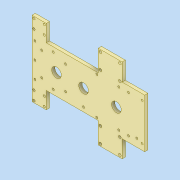
# Autodesk Inventor part: 底盘4.0
Saved by Autodesk Inventor 2019 (Build 230136000, 136)
## iProperties
Created: 2020-11-02
Part Number: 底盘4.0
Material: 尼龙 6/6
Document SubType Name: Modeling
Designer: Wang Hua
Density: 1.13 g/cm^3
Appearance: 尼龙 6
Mass: 59.1636 g
Surface Area: 303.115 cm^2
Volume: 52.3571 cm^3
Author: Wang Hua
Autodesk Inventor part; units mm, degrees
ref_plane "YZ Plane" through (0, 0, 0) normal (1, 0, 0) x (0, 1, 0)
ref_plane "XZ Plane" through (0, 0, 0) normal (0, 1, 0) x (-1, 0, 0)
ref_plane "XY Plane" through (0, 0, 0) normal (0, 0, 1) x (1, 0, 0)
sketch "草图1" plane through (0, 0, 0) normal (0, 0, 1) x (1, 0, 0)
  line L0 (-144.4444, 0) -> (-144.4444, 58)
  line L1 (-144.4444, 58) -> (-122.4444, 58)
  line L2 (-122.4444, 58) -> (-122.4444, 32)
  line L3 (-122.4444, 32) -> (-41.9444, 32)
  line L4 (-41.9444, 32) -> (-41.9444, 65)
  line L5 (-41.9444, 65) -> (-4.9444, 65)
  line L6 (-4.9444, 65) -> (-4.9444, 38)
  line L7 (-4.9444, 38) -> (30.0556, 38)
  line L8 (30.0556, 38) -> (30.0556, 0)
  line L9 (0, 0) -> (-166.6667, 0) construction
  line L10 (-144.4444, 0) -> (-144.4444, -58)
  line L11 (-144.4444, -58) -> (-122.4444, -58)
  line L12 (-122.4444, -58) -> (-122.4444, -32)
  line L13 (-122.4444, -32) -> (-41.9444, -32)
  line L14 (-41.9444, -32) -> (-41.9444, -65)
  line L15 (-41.9444, -65) -> (-4.9444, -65)
  line L16 (-4.9444, -65) -> (-4.9444, -38)
  line L17 (-4.9444, -38) -> (30.0556, -38)
  line L18 (30.0556, -38) -> (30.0556, 0)
  circle A0 centre (-106.5528, 0) radius 7.5
  circle A1 centre (-64.5976, 0) radius 7.5
  point P0 (-141.4444, -54)
  point P1 (-127.4444, -54)
  point P2 (-27.9137, -54)
  point P3 (-14.1378, -54)
  point P4 (-112.1204, -28)
  point P5 (-64.5976, -28)
  point P6 (-89.6514, -28)
  point P7 (-127.4444, -38)
  point P8 (-141.4444, -38)
  point P9 (-27.9137, -38)
  point P10 (-14.3619, -38)
  point P11 (-141.4444, 54)
  point P12 (-127.4444, 54)
  point P13 (-127.4444, 38)
  point P14 (-141.4444, 38)
  point P15 (-27.9137, 54)
  point P16 (-27.9137, 38)
  point P17 (-14.1378, 54)
  point P18 (-14.3619, 38)
  point P19 (-64.5976, 28)
  point P20 (-89.6514, 28)
  point P21 (-112.1204, 28)
  point P22 (-133.4444, 58)
  point P23 (-23.4444, 65)
  dimension "d0" = 22
  dimension "d1" = 37
  dimension "d3" = 32
  dimension "d4" = 38
  dimension "d5" = 35
  dimension "d6" = 58
  dimension "d7" = 15
  dimension "d8" = 15
  dimension "d29" = 28
  dimension "d30" = 28
  dimension "d31" = 28
  dimension "d36" = 110
  dimension "d96" = 33
  constraints: 38 end point, 19 symmetric about line, 5 perpendicular, 4 point on line, 2 centre point, 2 midpoint, 2 vertical, 1 horizontal
  measures "d0" distance of L0.end L1.end
  measures "d1" distance of L4.end L5.end
  measures "d3" distance between parallel lines of L9 L3
  measures "d4" distance between parallel lines of L9 L7
  measures "d5" distance of L6.end L7.end
  measures "d6" distance of L0.start L0.end
  measures "d7" diameter of A0
  measures "d8" diameter of A1
  measures "d29" distance from line of L9 point (-112.12, 28)
  measures "d30" distance from line of L9 point (-89.651, 28)
  measures "d31" distance from line of L9 point (-64.598, 28)
  measures "d36" horizontal distance of point (-23.444, 65) point (-133.444, 58)
  measures "d96" distance between parallel lines of L5 L3
extrude "拉伸1" add sketch "草图1" along normal blind 5
sketch "草图2" plane through (0, 0, 5) normal (0, 0, 1) x (1, 0, 0)
  circle A0 centre (-64.5976, 0) radius 7.5 construction
  circle A1 centre (-106.5528, 0) radius 7.5 construction
  line L0 (-144.4444, -58) -> (-144.4444, 58) construction
  line L1 (-144.4444, 58) -> (-122.4444, 58) construction
  line L2 (-122.4444, 58) -> (-122.4444, 32) construction
  line L3 (-122.4444, 32) -> (-41.9444, 32) construction
  line L4 (-41.9444, 32) -> (-41.9444, 65) construction
  line L5 (-41.9444, 65) -> (-4.9444, 65) construction
  line L6 (-4.9444, 65) -> (-4.9444, 38) construction
  line L7 (-4.9444, 38) -> (30.0556, 38) construction
  line L8 (30.0556, 38) -> (30.0556, -38) construction
  line L9 (30.0556, -38) -> (-4.9444, -38) construction
  line L10 (-4.9444, -38) -> (-4.9444, -65) construction
  line L11 (-4.9444, -65) -> (-41.9444, -65) construction
  line L12 (-41.9444, -65) -> (-41.9444, -32) construction
  line L13 (-41.9444, -32) -> (-122.4444, -32) construction
  line L14 (-122.4444, -32) -> (-122.4444, -58) construction
  line L15 (-122.4444, -58) -> (-144.4444, -58) construction
  line L16 (-164.7255, 0) -> (-80.9793, 0) construction
  point P0 (0, 0)
  point P1 (-141.4444, 55)
  point P2 (-125.4444, 55)
  point P3 (-38.4444, 61.5)
  point P4 (-8.4444, 61.5)
  point P5 (-38.4444, 37.5)
  point P6 (-8.4444, 37.5)
  point P7 (-125.4444, 41)
  point P8 (-141.4444, 41)
  point P9 (-141.4444, -55)
  point P10 (-125.4444, -55)
  point P11 (-38.4444, -61.5)
  point P12 (-8.4444, -61.5)
  point P13 (-38.4444, -37.5)
  point P14 (-8.4444, -37.5)
  point P15 (-125.4444, -41)
  point P16 (-141.4444, -41)
  dimension "d32" = 3
  dimension "d33" = 3
  dimension "d34" = 16
  dimension "d37" = 3
  dimension "d38" = 14
  dimension "d39" = 3
  dimension "d40" = 14
  dimension "d42" = 30
  dimension "d43" = 30
  dimension "d44" = 24
  dimension "d45" = 3.5
  dimension "d46" = 3.5
  dimension "d47" = 3.5
  dimension "d95" = 16
  constraints: 8 symmetric about line, 2 end point, 1 horizontal
  measures "d32" distance from line of L1 point (-125.444, 55)
  measures "d33" distance from line of L1 point (-141.444, 55)
  measures "d34" distance of point (-125.444, 55) point (-141.444, 55)
  measures "d37" distance from line of L0 point (-141.444, 55)
  measures "d38" distance of point (-141.444, 55) point (-141.444, 41)
  measures "d39" distance from line of L0 point (-141.444, 41)
  measures "d40" distance of point (-125.444, 55) point (-125.444, 41)
  measures "d42" distance of point (-8.444, 61.5) point (-38.444, 61.5)
  measures "d43" distance of point (-8.444, 37.5) point (-38.444, 37.5)
  measures "d44" distance of point (-38.444, 61.5) point (-38.444, 37.5)
  measures "d45" distance from line of L5 point (-38.444, 61.5)
  measures "d46" distance from line of L4 point (-38.444, 37.5)
  measures "d47" distance from line of L4 point (-38.444, 61.5)
  measures "d95" distance of point (-141.444, 41) point (-125.444, 41)
hole "孔2" at (-141.4444, 55, 5) at (-125.4444, 55, 5) at (-125.4444, 41, 5) at (-141.4444, 41, 5) at (-141.4444, -41, 5) at (-125.4444, -41, 5) at (-125.4444, -55, 5) at (-141.4444, -55, 5) direction (0, 0, -1) diameter 3.6 end through all
sketch "草图3" plane through (0, 0, 5) normal (0, 0, 1) x (1, 0, 0)
  circle A0 centre (-125.4444, -55) radius 1.8 construction
  circle A1 centre (-141.4444, -55) radius 1.8 construction
  circle A2 centre (-125.4444, 41) radius 1.8 construction
  circle A3 centre (-141.4444, 55) radius 1.8 construction
  circle A4 centre (-125.4444, 55) radius 1.8 construction
  circle A5 centre (-141.4444, 41) radius 1.8 construction
  circle A6 centre (-141.4444, -41) radius 1.8 construction
  circle A7 centre (-125.4444, -41) radius 1.8 construction
  circle A8 centre (-64.5976, 0) radius 7.5 construction
  circle A9 centre (-106.5528, 0) radius 7.5 construction
  line L0 (-144.4444, 58) -> (-144.4444, -58) construction
  line L1 (-144.4444, -58) -> (-122.4444, -58) construction
  line L2 (-122.4444, -58) -> (-122.4444, -32) construction
  line L3 (-122.4444, -32) -> (-41.9444, -32) construction
  line L4 (-41.9444, -32) -> (-41.9444, -65) construction
  line L5 (-41.9444, -65) -> (-4.9444, -65) construction
  line L6 (-4.9444, -65) -> (-4.9444, -38) construction
  line L7 (-4.9444, -38) -> (30.0556, -38) construction
  line L8 (30.0556, -38) -> (30.0556, 38) construction
  line L9 (30.0556, 38) -> (-4.9444, 38) construction
  line L10 (-4.9444, 38) -> (-4.9444, 65) construction
  line L11 (-4.9444, 65) -> (-41.9444, 65) construction
  line L12 (-41.9444, 65) -> (-41.9444, 32) construction
  line L13 (-41.9444, 32) -> (-122.4444, 32) construction
  line L14 (-122.4444, 32) -> (-122.4444, 58) construction
  line L15 (-122.4444, 58) -> (-144.4444, 58) construction
  line L16 (0, 0) -> (-184.5407, 0) construction
  point P0 (-139.9444, 25.8646)
  point P1 (-139.9444, 10.9473)
  point P2 (-108.7515, 25.8646)
  point P3 (-89.9847, 25.8646)
  point P4 (-70.7366, 25.8646)
  point P5 (-139.9444, -25.8646)
  point P6 (-139.9444, -10.9473)
  point P7 (-108.7515, -25.8646)
  point P8 (-89.9847, -25.8646)
  point P9 (-70.7366, -25.8646)
  point P10 (-139.9444, 0)
  constraints: 5 symmetric about line, 2 end point, 1 horizontal, 1 point on line
hole "孔3" at (-139.9444, 25.8646, 5) at (-139.9444, -25.8646, 5) at (-139.9444, 0, 5) direction (0, 0, -1) diameter 3.2 end through all
sketch "草图4" plane through (0, 0, 5) normal (0, 0, 1) x (1, 0, 0)
  circle A0 centre (-13.8026, 0) radius 7.5
  line L0 (0, 0) -> (-54.2498, 0) construction
  line L1 (-144.4444, 58) -> (-144.4444, -58) construction
  line L2 (30.0556, -38) -> (30.0556, 38) construction
  point P0 (-19.9444, 18.5)
  point P1 (17.0556, 18.5)
  point P2 (9.0556, 35)
  point P3 (-19.9444, -18.5)
  point P4 (17.0556, -18.5)
  point P5 (9.0556, -35)
  point P6 (-65.2677, 13.1999)
  point P7 (-65.2677, -14.7401)
  dimension "d62" = 15
  dimension "d67" = 37
  dimension "d68" = 50
  dimension "d69" = 18.5
  dimension "d70" = 35
  dimension "d71" = 21
  dimension "d94" = 27.94
  constraints: 3 symmetric about line, 2 end point, 1 centre point, 1 horizontal
  measures "d62" diameter of A0
  measures "d67" distance of point (17.056, 18.5) point (-19.944, 18.5)
  measures "d68" distance from line of L2 point (-19.944, 18.5)
  measures "d69" distance from line of L0 point (-19.944, 18.5)
  measures "d70" distance from line of L0 point (9.056, 35)
  measures "d71" distance from line of L2 point (9.056, 35)
  measures "d94" distance of point (-65.268, -14.74) point (-65.268, 13.2)
extrude "拉伸2" cut sketch "草图4" against normal through all
sketch "草图5" plane through (0, 0, 5) normal (0, 0, 1) x (1, 0, 0)
  line L0 (30.0556, -38) -> (30.0556, 38) projected
  line L1 (0, 0) -> (-47.6944, 0) construction
  point P0 (26.0556, 29)
  point P1 (-43.9444, 29)
  point P2 (-43.7151, 20)
  point P3 (26.0556, -29)
  point P4 (-43.9444, -29)
  point P5 (-43.7151, -20)
  dimension "d81" = 70
  dimension "d83" = 4
  dimension "d84" = 29
  dimension "d85" = 20
  dimension "d86" = 29
  constraints: 3 symmetric about line, 2 end point, 1 horizontal
  measures "d81" distance of point (-43.944, 29) point (26.056, 29)
  measures "d83" distance from line of L0 point (26.056, 29)
  measures "d84" vertical distance of L1.start point (26.056, 29)
  measures "d85" distance from line of L1 point (-43.715, 20)
  measures "d86" distance from line of L1 point (-43.944, 29)
hole "孔5" at (-43.9444, 29, 5) at (-43.9444, -29, 5) at (26.0556, 29, 5) at (26.0556, -29, 5) direction (0, 0, -1) diameter 3.2 end through all
hole "孔6" at (-38.4444, 61.5, 5) at (-8.4444, 61.5, 5) at (-38.4444, 37.5, 5) at (-8.4444, 37.5, 5) at (-38.4444, -37.5, 5) at (-8.4444, -37.5, 5) at (-8.4444, -61.5, 5) at (-38.4444, -61.5, 5) direction (0, 0, -1) diameter 4.2 end through all
sketch "草图6" plane through (0, 0, 5) normal (0, 0, 1) x (1, 0, 0)
  line L0 (-144.4444, 58) -> (-144.4444, -58) projected
  line L1 (0, 0) -> (-40.7503, 0) construction
  point P0 (-129.4444, 18.5)
  point P1 (-92.4444, 18.5)
  point P2 (-129.4444, -18.5)
  point P3 (-92.4444, -18.5)
  dimension "d104" = 15
  dimension "d105" = 37
  dimension "d106" = 18.5
  dimension "d107" = 18.5
  constraints: 2 end point, 2 symmetric about line, 1 horizontal
  measures "d104" distance from line of L0 point (-129.444, 18.5)
  measures "d105" distance of point (-129.444, 18.5) point (-92.444, 18.5)
  measures "d106" distance from line of L1 point (-92.444, 18.5)
  measures "d107" distance from line of L1 point (-129.444, 18.5)
hole "孔7" at (-129.4444, 18.5, 5) at (-92.4444, 18.5, 5) at (-129.4444, -18.5, 5) at (-92.4444, -18.5, 5) direction (0, 0, -1) diameter 3.2 end through all
sketch "草图7" plane through (0, 0, 5) normal (0, 0, 1) x (1, 0, 0)
  point P0 (0, 0)
  point P1 (11.1767, 22.7515)
  point P2 (17.9767, -25.8485)
  point P3 (-62.1233, 22.7515)
  point P4 (-64.6233, -25.2485)
  dimension "d115" = 48.6
  dimension "d116" = 6.8
  dimension "d117" = 73.3
  dimension "d118" = 48
  dimension "d119" = 2.5
  measures "d115" vertical distance of point (17.977, -25.849) point (11.177, 22.751)
  measures "d116" horizontal distance of point (17.977, -25.849) point (11.177, 22.751)
  measures "d117" distance of point (11.177, 22.751) point (-62.123, 22.751)
  measures "d118" vertical distance of point (-64.623, -25.249) point (-62.123, 22.751)
  measures "d119" horizontal distance of point (-62.123, 22.751) point (-64.623, -25.249)
hole "孔8" at (-64.6233, -25.2485, 5) at (17.9767, -25.8485, 5) direction (0, 0, -1) diameter 3.2 end through all
sketch "草图8" plane through (0, 0, 5) normal (0, 0, 1) x (1, 0, 0)
  line L0 (30.0556, 38) -> (-4.9444, 38) projected
  line L1 (0, 0) -> (93.7016, 0) construction
  line L2 (30.0556, -38) -> (30.0556, 38) projected
  line L3 (-41.9444, 32) -> (-122.4444, 32) projected
  point P0 (5.0556, 29)
  point P1 (-9.9444, 29)
  point P2 (5.0556, -29)
  point P3 (-9.9444, -29)
  point P4 (-111.5097, 25)
  point P5 (-111.5097, -25)
  dimension "d127" = 15
  dimension "d128" = 9
  dimension "d129" = 9
  dimension "d137" = 25
  dimension "d138" = 7
  constraints: 3 symmetric about line, 2 end point, 1 horizontal
  measures "d127" distance of point (5.056, 29) point (-9.944, 29)
  measures "d128" distance from line of point (5.056, 29) L0
  measures "d129" distance from line of L0 point (-9.944, 29)
  measures "d137" distance from line of L2 point (5.056, 29)
  measures "d138" distance from line of point (-111.51, 25) L3
hole "孔9" at (5.0556, 29, 5) at (-9.9444, 29, 5) at (-9.9444, -29, 5) at (5.0556, -29, 5) at (-111.5097, 25, 5) at (-111.5097, -25, 5) direction (0, 0, -1) diameter 3.2 end through all
